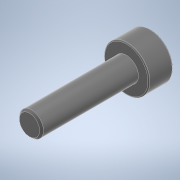
# Autodesk Inventor part: DIN 912 M2.5 8 mm
Saved by Autodesk Inventor 2022 (Build 260153000, 153)
## iProperties
Created: 2021-10-06
Part Number: DIN 912 M2.5 8 mm
Material: Generic
Document SubType Name: Modeling
Designer: Administrator
Density: 1 g/cm^3
Appearance: Smooth - Black
Mass: 0.0728763 g
Surface Area: 1.4959 cm^2
Volume: 0.0728763 cm^3
Title: DIN 912 M2.5 8 mm
Author: Administrator
Autodesk Inventor part; units mm, degrees
ref_plane "YZ Plane" through (0, 0, 0) normal (1, 0, 0) x (0, 1, 0)
ref_plane "XZ Plane" through (0, 0, 0) normal (0, 1, 0) x (-1, 0, 0)
ref_plane "Work Plane1" through (0, 0, -2.5) normal (0, 0, 1) x (1, 0, 0)
sketch "Sketch1" plane through (0, 0, -2.5) normal (0, 0, 1) x (1, 0, 0)
  circle A0 centre (0, 0) radius 2.34
  constraints: 1 centre point
extrude "Extrusion3" add sketch "Sketch1" along normal blind 2.5
sketch "Sketch2" plane through (0, 0, 0) normal (0, 0, 1) x (1, 0, 0)
  circle A0 centre (0, 0) radius 1.25
  constraints: 1 centre point
extrude "Extrusion2" add sketch "Sketch2" along normal blind 10
sketch "Sketch3" plane through (0, 0, -2.5) normal (0, 0, 1) x (1, 0, 0)
  line L0 (0.5947, -1.03) -> (-0.5947, -1.03)
  line L1 (0.5947, 1.03) -> (1.1893, 0)
  line L2 (-0.5947, -1.03) -> (-1.1893, 0)
  line L3 (-1.1893, 0) -> (-0.5947, 1.03)
  line L4 (1.1893, 0) -> (0.5947, -1.03)
  line L5 (-0.5947, 1.03) -> (0.5947, 1.03)
  constraints: 12 end point, 5 equal length, 2 horizontal
extrude "Extrusion1" cut sketch "Sketch3" along normal blind 2.5
fillet "Fillet1" radius 0.1 2 edges at (-2.34, 0, 0) (-2.34, 0, -2.5)
chamfer "Chamfer1" distance 0.2 angle 45 1 edges at (-1.25, 0, 10)
body "Solid3"
